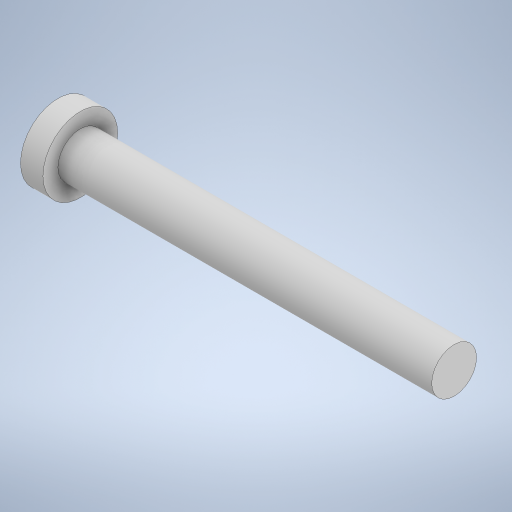
# Autodesk Inventor part: Part6
Saved by Autodesk Inventor 2024 (Build 280153000, 153)
## iProperties
Created: 2023-12-18
Part Number: Part6
Material: Generic
Document SubType Name: Modeling
Designer: SAHITYA
Density: 1 g/cm^3
Appearance: Default
Author: SAHITYA
Autodesk Inventor part; units mm, degrees
ref_plane "YZ Plane" through (0, 0, 0) normal (1, 0, 0) x (0, 1, 0)
ref_plane "XZ Plane" through (0, 0, 0) normal (0, 1, 0) x (-1, 0, 0)
ref_plane "XY Plane" through (0, 0, 0) normal (0, 0, 1) x (1, 0, 0)
sketch "Sketch1" plane through (0, 0, 0) normal (0, 1, 0) x (-1, 0, 0)
  line L0 (16.9868, 0.0221) -> (-8.0132, 0.0221)
  line L1 (-8.0132, 0.0221) -> (-8.0132, -1.4779)
  line L2 (-8.0132, -1.4779) -> (16.9868, -1.4779)
  line L3 (16.9868, -1.4779) -> (16.9868, 0.0221)
  line L4 (16.9868, 0.0221) -> (16.9868, -2.4779)
  line L5 (16.9868, -2.4779) -> (18.4868, -2.4779)
  line L6 (18.4868, -2.4779) -> (18.4868, 0.0221)
  line L7 (18.4868, 0.0221) -> (16.9868, 0.0221)
  dimension "d3" = 25
  dimension "d4" = 1.5
  dimension "d5" = 2.5
  dimension "d6" = 1.5
  constraints: 16 end point, 6 perpendicular, 2 point on line, 1 horizontal
  measures "d3" distance of L0.start L0.end
  measures "d4" distance of L0.end L1.end
  measures "d5" distance of L0.start L4.end
  measures "d6" distance of L4.end L5.end
revolve "Revolution1" add sketch "Sketch1" angle 360 about axis through (-16.9868, 0, 0.0221) along (1, 0, 0)
body "Solid1"
